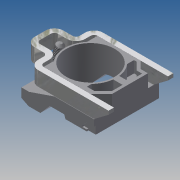
# Autodesk Inventor part: Mounting Collar
Saved by Autodesk Inventor 2014 (Build 180170000, 170)
## iProperties
Created: 2014-11-11
Part Number: Mounting Collar
Material: Generic
Description: Pushbutton Mounting Collar, Type: XB4, Size: 22mm
Document SubType Name: Modeling
Designer: David
Density: 1 g/cm^3
Appearance: Default
Author: David
Autodesk Inventor part; units mm, degrees
ref_plane "YZ Plane" through (0, 0, 0) normal (1, 0, 0) x (0, 1, 0)
ref_plane "XZ Plane" through (0, 0, 0) normal (0, 1, 0) x (-1, 0, 0)
ref_plane "XY Plane" through (0, 0, 0) normal (0, 0, 1) x (1, 0, 0)
sketch "Sketch1" plane through (0, 0, 0) normal (0, 1, 0) x (-1, 0, 0)
  line L0 (-22.225, 11.8745) -> (8.763, 11.8745)
  line L1 (10.287, 10.3505) -> (10.287, 7.874)
  line L2 (14.224, 3.937) -> (18.288, 3.937)
  line L3 (19.812, 2.413) -> (19.812, -2.413)
  line L4 (18.288, -3.937) -> (14.224, -3.937)
  line L5 (10.287, -7.874) -> (10.287, -10.3505)
  line L6 (8.763, -11.8745) -> (-22.225, -11.8745)
  line L7 (-22.225, -11.8745) -> (-22.225, -14.2875)
  line L8 (-22.225, -14.2875) -> (8.763, -14.2875)
  line L9 (12.7, -10.3505) -> (12.7, -7.874)
  line L10 (14.224, -6.35) -> (18.288, -6.35)
  line L11 (22.225, -2.413) -> (22.225, 2.413)
  line L12 (18.288, 6.35) -> (14.224, 6.35)
  line L13 (12.7, 7.874) -> (12.7, 10.3505)
  line L14 (8.763, 14.2875) -> (-22.225, 14.2875)
  line L15 (-22.225, 14.2875) -> (-22.225, 11.8745)
  line L16 (0, -21.144031) -> (0, 21.144031) construction
  line L17 (-31.278076, 0) -> (32.093455, 0) construction
  arc A0 (10.287, 10.3505) -> (8.763, 11.8745) centre (8.763, 10.3505) ccw
  arc A1 (14.224, -6.35) -> (12.7, -7.874) centre (14.224, -7.874) ccw
  arc A2 (8.763, -11.8745) -> (10.287, -10.3505) centre (8.763, -10.3505) ccw
  arc A3 (12.7, 7.874) -> (14.224, 6.35) centre (14.224, 7.874) ccw
  arc A4 (19.812, 2.413) -> (18.288, 3.937) centre (18.288, 2.413) ccw
  arc A5 (18.288, -3.937) -> (19.812, -2.413) centre (18.288, -2.413) ccw
  arc A6 (12.7, 10.3505) -> (8.763, 14.2875) centre (8.763, 10.3505) ccw
  arc A7 (8.763, -14.2875) -> (12.7, -10.3505) centre (8.763, -10.3505) ccw
  arc A8 (14.224, -3.937) -> (10.287, -7.874) centre (14.224, -7.874) ccw
  arc A9 (18.288, -6.35) -> (22.225, -2.413) centre (18.288, -2.413) ccw
  arc A10 (22.225, 2.413) -> (18.288, 6.35) centre (18.288, 2.413) ccw
  arc A11 (10.287, 7.874) -> (14.224, 3.937) centre (14.224, 7.874) ccw
  point P0 (0, 0)
  point P1 (22.225, 6.35)
  point P2 (12.7, 6.35)
  dimension "d0" = 22.225
  dimension "d1" = 2.413
  dimension "d2" = 2.413
  dimension "d3" = 2.413
  dimension "d4" = 2.413
  dimension "d5" = 44.45
  dimension "d6" = 12.7
  dimension "d7" = 9.525
  dimension "d8" = 28.575
  dimension "d9" = 1.524
  dimension "d10" = 3.937
  constraints: 32 end point, 24 point on circle, 24 tangent, 12 centre point, 10 equal radius, 9 parallel, 4 point on line, 3 collinear, 3 equal length, 3 perpendicular, 2 horizontal, 3 other
  measures "d0" distance from line of L11 point (0, 0)
  measures "d1" distance of L14.end L0.start
  measures "d2" distance between parallel lines of L1 L13
  measures "d3" distance between parallel lines of L11 L3
  measures "d4" distance between parallel lines of L2 L12
  measures "d5" distance between parallel lines of L11 L15
  measures "d6" distance between parallel lines of L10 L12
  measures "d7" distance of point (22.225, 6.35) point (12.7, 6.35)
  measures "d8" distance between parallel lines of L8 L14
  measures "d9" radius of A0
  measures "d10" radius of A6
extrude "Extrusion1" add sketch "Sketch1" against normal blind 6.35
sketch "Sketch2" plane through (-8.763, 0, 14.2875) normal (0, 0, 1) x (1, 0, 0)
  line L0 (0, 0) -> (30.988, 0) projected
  line L1 (30.988, -6.35) -> (0, -6.35) projected
  line L2 (30.988, 0) -> (30.988, -6.35) projected
  line L3 (30.988, -1.5875) -> (24.638, -6.35)
  line L4 (24.638, -6.35) -> (30.988, -6.35)
  line L5 (30.988, -1.5875) -> (30.988, -6.35)
  point P0 (8.763, 0)
  dimension "d13" = 1.5875
  dimension "d14" = 6.35
  constraints: 6 end point, 2 collinear, 2 point on line
  measures "d13" distance from line of L3.start L0
  measures "d14" distance of L3.end L1.start
extrude "Extrusion2" cut sketch "Sketch2" against normal through all
sketch "Sketch3" plane through (0, 0, 0) normal (0, 1, 0) x (-1, 0, 0)
  circle A0 centre (0, 0) radius 10.668
  line L0 (-22.225, 11.8745) -> (8.763, 11.8745) construction
  arc A1 (10.287, 10.3505) -> (8.763, 11.8745) centre (8.763, 10.3505) ccw construction
  line L1 (10.287, 10.3505) -> (10.287, 7.874) construction
  arc A2 (10.287, 7.874) -> (14.224, 3.937) centre (14.224, 7.874) ccw construction
  line L2 (14.224, 3.937) -> (18.288, 3.937) construction
  arc A3 (19.812, 2.413) -> (18.288, 3.937) centre (18.288, 2.413) ccw construction
  line L3 (19.812, 2.413) -> (19.812, -2.413) construction
  arc A4 (18.288, -3.937) -> (19.812, -2.413) centre (18.288, -2.413) ccw construction
  line L4 (18.288, -3.937) -> (14.224, -3.937) construction
  arc A5 (14.224, -3.937) -> (10.287, -7.874) centre (14.224, -7.874) ccw construction
  line L5 (10.287, -7.874) -> (10.287, -10.3505) construction
  arc A6 (8.763, -11.8745) -> (10.287, -10.3505) centre (8.763, -10.3505) ccw construction
  line L6 (8.763, -11.8745) -> (-22.225, -11.8745) construction
  line L7 (-22.225, -11.8745) -> (-22.225, -14.2875) construction
  line L8 (-22.225, -14.2875) -> (8.763, -14.2875) construction
  arc A7 (8.763, -14.2875) -> (12.7, -10.3505) centre (8.763, -10.3505) ccw construction
  line L9 (12.7, -10.3505) -> (12.7, -7.874) construction
  arc A8 (14.224, -6.35) -> (12.7, -7.874) centre (14.224, -7.874) ccw construction
  line L10 (14.224, -6.35) -> (18.288, -6.35) construction
  arc A9 (18.288, -6.35) -> (22.225, -2.413) centre (18.288, -2.413) ccw construction
  line L11 (22.225, -2.413) -> (22.225, 2.413) construction
  arc A10 (22.225, 2.413) -> (18.288, 6.35) centre (18.288, 2.413) ccw construction
  line L12 (18.288, 6.35) -> (14.224, 6.35) construction
  arc A11 (12.7, 7.874) -> (14.224, 6.35) centre (14.224, 7.874) ccw construction
  line L13 (12.7, 7.874) -> (12.7, 10.3505) construction
  arc A12 (12.7, 10.3505) -> (8.763, 14.2875) centre (8.763, 10.3505) ccw construction
  line L14 (8.763, 14.2875) -> (-22.225, 14.2875) construction
  line L15 (-22.225, 14.2875) -> (-22.225, 11.8745) construction
  line L16 (8.763, 11.8491) -> (8.763, 7.279414)
  arc A13 (8.763, -7.279414) -> (8.763, 7.279414) centre (0, 0) ccw
  line L17 (8.763, -7.279414) -> (8.763, -11.8491)
  line L18 (8.763, -11.8491) -> (-10.287, -11.8491)
  line L19 (-10.287, -11.8491) -> (-13.462, -8.6741)
  line L20 (-13.462, -8.6741) -> (-16.637, -8.6741)
  line L21 (-16.637, -8.6741) -> (-16.637, 7.0866)
  line L22 (-16.637, 7.0866) -> (-11.8745, 11.8491)
  line L23 (-11.8745, 11.8491) -> (8.763, 11.8491)
  dimension "d17" = 21.336
  dimension "d18" = 0.0254
  dimension "d19" = 0.0254
  dimension "d20" = 19.05
  dimension "d21" = 6.35
  dimension "d22" = 3.175
  dimension "d23" = 3.175
  dimension "d24" = 4.7625
  dimension "d25" = 4.7625
  constraints: 16 end point, 3 parallel, 2 centre point, 2 coincident, 2 collinear, 2 perpendicular, 2 point on circle, 1 point on line
  measures "d17" diameter of A0
  measures "d18" distance between parallel lines of L23 L0
  measures "d19" distance between parallel lines of L6 L18
  measures "d20" distance of L17.end L18.end
  measures "d21" distance from line of L18.end L21
  measures "d22" distance of L19.end L20.end
  measures "d23" horizontal distance of L18.end L19.end
  measures "d24" horizontal distance of L21.end L22.end
  measures "d25" horizontal distance of L21.end L22.end
extrude "Extrusion3" add sketch "Sketch3" against normal blind 6.731
sketch "Sketch4" plane through (0, 0, 0) normal (0, 1, 0) x (1, 0, 0)
  circle A0 centre (0, 0) radius 10.668
  line L0 (-8.763, -11.8491) -> (-8.763, -7.279414)
  line L1 (10.287, 11.8491) -> (13.462, 8.6741)
  line L2 (-8.763, 7.279414) -> (-8.763, 11.8491)
  line L3 (8.54045, 10.629308) -> (8.54045, 7.590505)
  arc A1 (11.347952, 1.333805) -> (8.54045, 7.590505) centre (0, 0) ccw
  line L4 (8.54045, 10.629308) -> (9.7312, 10.629308)
  line L5 (9.7312, 10.629308) -> (13.119786, 7.240722)
  line L6 (13.119786, 7.240722) -> (15.474695, 7.240722)
  line L7 (15.474695, 7.240722) -> (15.474695, 1.333805)
  line L8 (15.474695, 1.333805) -> (11.347952, 1.333805)
  line L9 (11.347952, -1.333805) -> (15.474695, -1.333805)
  line L10 (15.474695, -1.333805) -> (15.474695, -6.101995)
  line L11 (15.474695, -6.101995) -> (11.696325, -9.880364)
  line L12 (11.696325, -9.880364) -> (8.303502, -9.880364)
  line L13 (8.303502, -9.880364) -> (8.303502, -7.849006)
  arc A2 (8.303502, -7.849006) -> (11.347952, -1.333805) centre (0, 0) ccw
  line L14 (31.115, 0) -> (-31.115, 0) construction
  constraints: 22 end point, 8 parallel, 4 perpendicular, 4 point on circle, 2 centre point, 2 coincident, 1 collinear, 1 concentric, 1 other
extrude "Extrusion4" cut sketch "Sketch4" against normal blind 5.08 contours L4 L5 L6 L7 L8 A1 L3 | L9 L10 L11 L12 L13 A2
sketch "Sketch5" plane through (-8.763, 0, 14.2875) normal (0, 0, 1) x (1, 0, 0)
  line L0 (0, 0) -> (30.988, 0)
  line L1 (24.638, -6.35) -> (0, -6.35)
  line L2 (24.638, -6.480135) -> (24.638, -12.7)
  line L3 (24.638, -12.7) -> (12.028577, -12.7)
  line L4 (12.028577, -12.7) -> (11.485563, -11.1125)
  line L5 (11.485563, -11.1125) -> (5.135563, -11.1125)
  line L6 (5.135563, -11.1125) -> (0.968375, -15.875)
  line L7 (0.968375, -15.875) -> (-4.191, -15.875)
  line L8 (-4.191, -15.875) -> (-7.366, -14.2875)
  line L9 (-7.366, -14.2875) -> (-7.366, -10.297086)
  line L10 (-7.366, -10.297086) -> (-3.983331, -10.297086)
  line L11 (-3.983331, -10.297086) -> (7.1755, -6.480135)
  line L12 (7.1755, -6.480135) -> (24.638, -6.480135)
  point P0 (8.763, 0)
  dimension "d30" = 12.7
  dimension "d32" = 1.5875
  dimension "d33" = 6.35
  dimension "d35" = 15.875
  dimension "d36" = 3.175
  dimension "d37" = 1.5875
  dimension "d40" = 17.4625
  constraints: 22 end point, 4 parallel, 4 perpendicular, 1 point on line
  measures "d30" distance between parallel lines of L3 L0
  measures "d32" vertical distance of L3.end L4.end
  measures "d33" distance of L4.end L5.end
  measures "d35" distance between parallel lines of L7 L0
  measures "d36" horizontal distance of L7.end L8.end
  measures "d37" vertical distance of L7.end L8.end
  measures "d40" distance of L11.end L2.start
extrude "Extrusion5" add sketch "Sketch5" against normal up to surface (28.575 mm away)
sketch "Sketch6" plane through (0, 0, 0) normal (0, 1, 0) x (1, 0, 0)
  circle A0 centre (0, 0) radius 10.668 projected
extrude "Extrusion6" cut sketch "Sketch6" against normal through all
sketch "Sketch7" plane through (0, -6.731, 0) normal (0, -1, 0) x (1, 0, 0)
  line L0 (-2.320903, -11.8491) -> (-2.320903, -10.412475)
  arc A0 (-2.320903, 10.412475) -> (-2.320903, -10.412475) centre (0, 0) ccw
  line L1 (-2.320903, 10.412475) -> (-2.320903, 11.8491)
  line L2 (-2.320903, 11.8491) -> (-8.763, 11.8491)
  line L3 (-8.763, 11.8491) -> (-8.763, 7.279414)
  arc A1 (-8.763, 7.279414) -> (-8.763, -7.279414) centre (0, 0) ccw
  line L4 (-8.763, -7.279414) -> (-8.763, -11.8491)
  line L5 (-8.763, -11.8491) -> (-2.320903, -11.8491)
extrude "Extrusion7" add sketch "Sketch7" along normal up to next
sketch "Sketch8" plane through (-12.954, -15.875, 14.2875) normal (0, -1, 0) x (1, 0, 0)
  line L0 (0, 0) -> (0, -28.575)
  line L1 (-18.161, -14.2875) -> (44.069, -14.2875) construction
  arc A0 (-6.539155, -12.986374) -> (-6.539155, -15.588626) centre (-4.062969, -14.2875) ccw
  line L2 (0, -7.288061) -> (-3.544945, -7.288061)
  line L3 (-3.544945, -7.288061) -> (-6.539155, -12.986374)
  line L4 (0, -21.286939) -> (-3.544945, -21.286939)
  line L5 (-3.544945, -21.286939) -> (-6.539155, -15.588626)
  line L6 (-3.175, 0) -> (-3.175, -28.575)
  line L7 (0, -7.288061) -> (0, -21.286939)
  dimension "d47" = 1.90925
  constraints: 10 end point, 3 symmetric about line, 2 point on circle, 2 point on line, 1 centre point, 1 collinear, 1 parallel, 1 tangent
  measures "d47" distance edge to line of A0 L6
extrude "Extrusion8" add sketch "Sketch8" against normal blind 6.35
sketch "Sketch9" plane through (-8.763, 0, 14.2875) normal (0, 0, 1) x (1, 0, 0)
  line L0 (-11.051187, -15.875) -> (-11.051187, -9.525) construction
  line L1 (-11.051187, -15.875) -> (-5.175086, -15.875)
  line L2 (-5.175086, -15.875) -> (-11.051187, -14.004039)
  line L3 (-11.051187, -14.004039) -> (-11.051187, -15.875)
  point P0 (8.763, 0)
  constraints: 6 end point, 1 collinear, 1 perpendicular, 1 point on line
extrude "Extrusion9" cut sketch "Sketch9" against normal through all
sketch "Sketch10" plane through (-13.938086, -15.875, -6.999439) normal (-0.303394, -0.9528652, 0) x (0.9528652, -0.303394, 0)
  circle A0 centre (-4.247184, 6.999439) radius 1.5875
  ellipse E0 centre (-3.231184, 6.999439) end of major axis (-6.166771, 6.999439) minor radius 2.797218 (-5.829859, 8.300565) -> (-5.829859, 5.698313) ccw
  point P0 (8.464737, 6.999439)
  dimension "d52" = 3.175
  dimension "d58" = 1.016
  constraints: 1 centre point, 1 other
  measures "d52" diameter of A0
  measures "d58" distance of point (-3.231, 6.999) A0.centre
extrude "Extrusion10" add sketch "Sketch10" against normal blind 16.51
chamfer "Chamfer1" distance 1.016 angle 45 1 edges at (-14.4887, 1.627, 0)
sketch "Sketch11" plane through (-13.938086, -15.875, -6.999439) normal (-0.303394, -0.9528652, 0) x (0.9528652, -0.303394, 0)
  circle A0 centre (-4.247184, 6.999439) radius 1.5875
  point P0 (8.464737, 6.999439)
extrude "Extrusion11" add sketch "Sketch11" along normal blind 4.7625
sketch "Sketch12" plane through (-19.429994, -19.12445, 0) normal (-0.303394, -0.9528652, 0) x (0.9528652, -0.303394, 0)
  circle A0 centre (0, 0) radius 1.5875 projected
  circle A1 centre (0, 0) radius 2.667
  point P0 (12.711921, 0)
  dimension "d61" = 5.334
  constraints: 1 centre point, 1 coincident
  measures "d61" diameter of A1
extrude "Extrusion12" add sketch "Sketch12" along normal blind 2.54 contours A0 | A1
fillet "Fillet1" radius 0.381 1 edges at (-22.7419, -20.7356, 0)
sketch "Sketch13" plane through (-20.200614, -21.544728, 0) normal (-0.303394, -0.9528652, 0) x (0.9528652, -0.303394, 0)
  circle A0 centre (0, 0) radius 2.286
  line L0 (-0.299851, 1.426002) -> (0.796309, 1.220362)
  line L1 (0.796309, 1.220362) -> (1.426002, 0.299851)
  line L2 (1.426002, 0.299851) -> (1.220362, -0.796309)
  line L3 (1.220362, -0.796309) -> (0.299851, -1.426002)
  line L4 (0.299851, -1.426002) -> (-0.796309, -1.220362)
  line L5 (-0.796309, -1.220362) -> (-1.426002, -0.299851)
  line L6 (-1.426002, -0.299851) -> (-1.220362, 0.796309)
  line L7 (-1.220362, 0.796309) -> (-0.299851, 1.426002)
  line L8 (-0.299851, 1.426002) -> (-0.796309, -1.220362)
  line L9 (-1.220362, 0.796309) -> (1.426002, 0.299851)
  line L10 (0.796309, 1.220362) -> (0.299851, -1.426002)
  line L11 (1.220362, -0.796309) -> (-1.426002, -0.299851)
  point P0 (12.711921, 0)
  constraints: 24 end point, 3 perpendicular, 1 coincident, 1 parallel, 17 other
sketch "Sketch13 outline for Extrusion13" plane through (-20.200614, -21.544728, 0) normal (-0.303394, -0.9528652, 0) x (0.9528652, -0.303394, 0)
  line L0 (0.44526, -0.6509) -> (1.220362, -0.796309)
  line L1 (1.220362, -0.796309) -> (1.426002, 0.299851)
  line L2 (1.426002, 0.299851) -> (0.6509, 0.44526)
  line L3 (0.6509, 0.44526) -> (0.796309, 1.220362)
  line L4 (0.796309, 1.220362) -> (-0.299851, 1.426002)
  line L5 (-0.299851, 1.426002) -> (-0.44526, 0.6509)
  line L6 (-0.44526, 0.6509) -> (-1.220362, 0.796309)
  line L7 (-1.220362, 0.796309) -> (-1.426002, -0.299851)
  line L8 (-1.426002, -0.299851) -> (-0.6509, -0.44526)
  line L9 (-0.6509, -0.44526) -> (-0.796309, -1.220362)
  line L10 (-0.796309, -1.220362) -> (0.299851, -1.426002)
  line L11 (0.299851, -1.426002) -> (0.44526, -0.6509)
extrude "Extrusion13" cut sketch "Sketch13 outline for Extrusion13" against normal blind 1.27 draft -15
thread "Thread1" size "5-40 UNC" class "2A" standard "ANSI Unified Screw Threads" full length
thread "Thread2" size "5-40 UNC" class "2A" standard "ANSI Unified Screw Threads" full length
sketch "Sketch14" plane through (-8.763, 0, 14.2875) normal (0, 0, 1) x (1, 0, 0)
  line L0 (24.638, -6.480135) -> (24.638, -12.7)
  line L1 (24.638, -12.7) -> (12.028577, -12.7)
  line L2 (24.638, -9.22894) -> (21.484097, -9.22894)
  line L3 (21.484097, -9.22894) -> (19.51026, -11.316215)
  line L4 (19.51026, -11.316215) -> (19.51026, -11.942835)
  line L5 (19.51026, -11.942835) -> (21.400251, -11.942835)
  line L6 (21.400251, -11.942835) -> (21.400251, -12.7)
  line L7 (21.400251, -12.7) -> (24.638, -12.7)
  line L8 (24.638, -12.7) -> (24.638, -9.22894)
  point P0 (8.763, 0)
  constraints: 14 end point, 3 perpendicular, 2 parallel, 2 point on line, 1 collinear
extrude "Extrusion14" cut sketch "Sketch14" against normal blind 0.762
ref_plane "Work Plane1" through (-8.763, 0, 9.3345) normal (0, 0, 1) x (1, 0, 0)
mirror "Mirror1" about plane through (-8.763, 0, 9.3345) normal (0, 0, 1) of "Extrusion14"
mirror "Mirror2" about plane through (0, 0, 0) normal (0, 0, 1) of "Extrusion14", "Mirror1"
equation "\"d2\" = d1"
equation "\"d3\" = d1"
equation "\"d4\" = d1"
equation "\"d25\" = d24"
body "Solid1"
